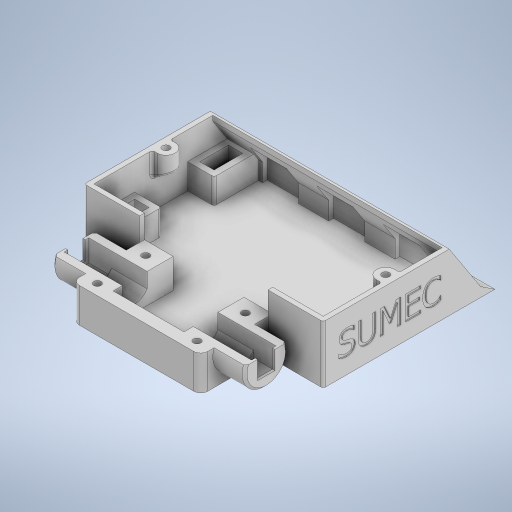
# Autodesk Inventor part: Tělo
Saved by Autodesk Inventor 2024 (Build 280153000, 153)
## iProperties
Created: 2023-04-15
Part Number: Tělo
Material: Všeobecné
Document SubType Name: Modeling
Designer: 42060
Density: 1 g/cm^3
Appearance: Výchozí
Author: 42060
Autodesk Inventor part; units mm, degrees
ref_plane "YZ Plane" through (0, 0, 0) normal (1, 0, 0) x (0, 1, 0)
ref_plane "XZ Plane" through (0, 0, 0) normal (0, 1, 0) x (-1, 0, 0)
ref_plane "XY Plane" through (0, 0, 0) normal (0, 0, 1) x (1, 0, 0)
sketch "Základ" plane through (0, 0, 0) normal (0, 0, 1) x (1, 0, 0)
  line L0 (0, 0) -> (49.75, 0)
  line L1 (49.75, 0) -> (49.75, -71.5)
  line L2 (49.75, -71.5) -> (26.75, -71.5)
  line L3 (26.75, -99.5) -> (0, -99.5)
  line L4 (0, -99.5) -> (0, 0)
  line L5 (0, -20) -> (47.75, -20)
  line L6 (47.75, -20) -> (47.75, -69.5)
  line L7 (47.75, -69.5) -> (14.75, -69.5)
  line L8 (14.75, -69.5) -> (14.75, -94.5)
  line L9 (14.75, -94.5) -> (0, -94.5)
  line L10 (26.75, -71.5) -> (26.75, -80.375)
  line L11 (26.75, -80.375) -> (26.75, -90.625)
  line L12 (26.75, -90.625) -> (26.75, -99.5)
  line L13 (26.75, -90.625) -> (14.75, -90.625)
  line L14 (26.75, -80.375) -> (14.75, -80.375)
  line L15 (26.75, -71.5) -> (26.75, -69.5)
  dimension "d0" = 49.75
  dimension "d1" = 99.5
  dimension "d3" = 2
  dimension "d5" = 28
  dimension "d14" = 10.25
  dimension "d15" = 12
  dimension "d16" = 5
  dimension "d17" = 23
  dimension "d18" = 2
  dimension "d19" = 20
  constraints: 32 end point, 8 perpendicular, 6 point on line, 3 horizontal, 2 collinear, 1 parallel, 1 vertical
  measures "d0" distance of L0.start L0.end
  measures "d1" distance between parallel lines of L3 L0
  measures "d3" distance between parallel lines of L1 L6
  measures "d5" distance of L2.end L3.start
  measures "d14" distance of L10.end L11.end
  measures "d15" distance between parallel lines of L8 L10
  measures "d16" distance between parallel lines of L9 L3
  measures "d17" distance between parallel lines of L1 L12
  measures "d18" distance between parallel lines of L2 L7
  measures "d19" distance between parallel lines of L0 L5
extrude "Podlaha" add sketch "Základ" along normal blind 2 contours L5 L6 L7 L8 L9 L4
extrude "Stěny" add sketch "Základ" along normal blind 24 contours L0 L1 L2 L15 L7 L6 L5 L4
extrude "Zadní stěny" add sketch "Základ" along normal blind 15 contours L9 L8 L13 L12 L3 L4 | L10 L14 L8 L7 L15
extrude "Stěna pod motorem" add sketch "Základ" along normal blind 5.25 contours L11 L13 L8 L14
sketch "Náčrt2" plane through (49.75, -71.5, 0) normal (1, 0, 0) x (0, 0, -1)
  line L0 (-2, 51.5) -> (-24, 51.5) projected
  line L1 (-2, 51.5) -> (-24, 51.5) projected
  line L2 (-24, 0) -> (-24, 71.5) projected
  line L3 (0, 71.5) -> (-24, 71.5) projected
  line L4 (0, 71.5) -> (0, 0) projected
  line L5 (-24, 52.5) -> (-4, 65.5)
  line L6 (-4, 65.5) -> (0, 71.5)
  dimension "d28" = 1
  dimension "d29" = 6
  dimension "d30" = 20
  constraints: 4 end point, 1 point on line
  measures "d28" distance from line of L5.start L0
  measures "d29" vertical distance of L3.start L5.end
  measures "d30" horizontal distance of L5.end L5.start
extrude "Rampa" cut sketch "Náčrt2" against normal through all
sketch "Náčrt3" plane through (0, -20, 2) normal (-1, 0, 0) x (0, 0, 1)
  line L0 (0, 0) -> (22, 0) projected
  line L1 (0, 0) -> (22, 0) projected
  line L2 (19.8687, 0) -> (7.5, 8.0396)
  line L3 (7.5, 8.0396) -> (0, 8.0396)
  line L4 (0, 8.0396) -> (0, 0)
  line L5 (22, 1) -> (2, 14) projected
  point P0 (-2, 20)
  point P1 (19.8687, 0)
  dimension "d34" = 7.5
  dimension "d37" = 2
  constraints: 6 end point, 1 horizontal, 1 parallel, 1 perpendicular, 1 point on line
  measures "d34" distance of L2.end L3.end
  measures "d37" distance between parallel lines of L2 L5
extrude "Přední rampa" cut sketch "Náčrt3" against normal up to surface (47.75 mm away)
sketch "Držák motoru" plane through (14.75, -94.5, 2) normal (-1, 0, 0) x (0, 0, 1)
  line L0 (3.25, 14.125) -> (13, 14.125) projected
  line L1 (3.25, 14.125) -> (3.25, 3.875) projected
  line L2 (3.25, 3.875) -> (13, 3.875) projected
  line L3 (6.13, 14.125) -> (12.37, 14.125)
  line L4 (12.37, 3.875) -> (6.13, 3.875)
  line L5 (3.25, 3.875) -> (13, 3.875) projected
  arc A0 (12.37, 3.875) -> (12.37, 14.125) centre (9.25, 9) ccw
  arc A1 (6.13, 14.125) -> (6.13, 3.875) centre (9.25, 9) ccw
  line L6 (15.25, 14.125) -> (15.25, 3.875) construction
  circle A2 centre (9.25, 9) radius 9
  line L7 (9.25, 18) -> (0, 18)
  line L8 (0, 0) -> (0, 82.5396) projected
  line L9 (0, 0) -> (13, 0) projected
  line L10 (13, -5) -> (13, 3.875) projected
  line L11 (0, 0) -> (13, 0) projected
  line L12 (0, 0) -> (13, 0) projected
  line L13 (12.37, 14.125) -> (12.37, 17.4419)
  line L14 (12.37, 3.875) -> (12.37, 0.5581)
  line L15 (12.37, 0.5581) -> (12.37, 0)
  line L16 (12.37, 17.4419) -> (12.37, 18)
  line L17 (12.37, 18) -> (9.25, 18)
  point P0 (-2, 94.5)
  point P1 (15.25, 9)
  point P2 (15.25, 9)
  point P3 (3.25, 9)
  point P4 (3.25, 9)
  point P5 (6.13, 3.875)
  point P6 (9.25, 0)
  point P7 (16.7333, 14)
  point P8 (16.7333, 4)
  point P9 (12.37, 0)
  dimension "d38" = 6
  dimension "d39" = 6
  dimension "d41" = 3
  dimension "d48" = 12
  constraints: 18 end point, 9 point on circle, 7 point on line, 4 tangent, 3 centre point, 3 coincident, 3 vertical, 2 horizontal alignment, 2 midpoint, 1 horizontal, 1 perpendicular
  measures "d38" radius of A0
  measures "d39" radius of A1
  measures "d41" radial gap between concentric circles of A2 A0
  measures "d48" distance between parallel lines of L1 L6
sketch "Náčrt10" plane through (14.75, -99.5, 0) normal (1, 0, 0) x (0, 0, -1)
  line L0 (-5.25, 8.875) -> (-15, 8.875) construction
  line L1 (-5.25, 8.875) -> (-17.25, 8.875) construction
  line L2 (-17.25, 8.875) -> (-17.25, 19.125) construction
  line L3 (-17.25, 19.125) -> (-5.25, 19.125) construction
  line L4 (-5.25, 19.125) -> (-5.25, 8.875) construction
  line L5 (-14.37, 8.875) -> (-8.13, 8.875)
  arc A0 (-8.13, 8.875) -> (-8.13, 19.125) centre (-11.25, 14) ccw
  line L6 (-14.37, 19.125) -> (-8.13, 19.125)
  arc A1 (-14.37, 5.5581) -> (-14.37, 22.4419) centre (-11.25, 14) ccw
  line L7 (-14.37, 8.875) -> (-14.37, 5.5581)
  line L8 (-14.37, 19.125) -> (-14.37, 22.4419)
  point P0 (0, 99.5)
  point P1 (-11.25, 19.125)
  point P2 (-11.25, 19.125)
  point P3 (-11.25, 8.875)
  point P4 (-11.25, 8.875)
  dimension "d79" = 12
  dimension "d80" = 6
  dimension "d81" = 18
  constraints: 16 end point, 5 point on line, 4 midpoint, 4 point on circle, 3 coincident, 2 centre point, 2 parallel, 2 perpendicular, 2 vertical alignment, 1 collinear, 1 horizontal, 1 horizontal alignment, 1 tangent
  measures "d79" distance between parallel lines of L4 L2
  measures "d80" radius of A0
  measures "d81" diameter of A1
extrude "Držák motoru (kulaté)" add sketch "Náčrt10" along normal blind 15
sketch "Náčrt11" plane through (29.75, -99.5, 0) normal (1, 0, 0) x (0, 0, -1)
  arc A0 (-8.13, 8.875) -> (-8.13, 19.125) centre (-11.25, 14) ccw projected
  circle A1 centre (-11.25, 14) radius 9
  line L0 (-17.25, 8.875) -> (-5.25, 8.875)
  line L1 (-5.25, 8.875) -> (-5.25, 19.125)
  line L2 (-5.25, 19.125) -> (-17.25, 19.125)
  line L3 (-17.25, 19.125) -> (-17.25, 8.875)
  line L4 (-17.25, 8.875) -> (-5.25, 19.125) construction
  line L5 (-5.25, 8.875) -> (-17.25, 19.125) construction
  line L6 (-14.37, 8.875) -> (-14.37, 5.5581) projected
  line L7 (-14.37, 22.4419) -> (-14.37, 19.125) projected
  point P0 (0, 99.5)
  dimension "d84" = 18
  constraints: 12 end point, 2 midpoint, 2 parallel, 1 centre point, 1 coincident, 1 horizontal, 1 horizontal alignment, 1 perpendicular, 1 tangent
  measures "d84" diameter of A1
extrude "Držák motoru (hranaté)" add sketch "Náčrt11" along normal blind 9.25 contours L0 L1 L2 L7 A1 L6
sketch "Náčrt7" plane through (0, 0, 2) normal (0, 0, 1) x (1, 0, 0)
  line L0 (0, -11.9604) -> (47.75, -11.9604) projected
  line L1 (0, -11.9604) -> (47.75, -11.9604) projected
  line L2 (0, 0) -> (0, -99.5) projected
  line L3 (0, -9.9604) -> (7.5, -9.9604)
  line L4 (7.5, -9.9604) -> (7.5, -16.9604)
  line L5 (7.5, -16.9604) -> (0, -16.9604)
  line L6 (0, -16.9604) -> (0, -9.9604)
  line L7 (20.125, -9.9604) -> (35.125, -9.9604)
  line L8 (35.125, -9.9604) -> (35.125, -16.9604)
  line L9 (35.125, -16.9604) -> (20.125, -16.9604)
  line L10 (20.125, -16.9604) -> (20.125, -9.9604)
  point P0 (27.625, -16.9604)
  point P1 (35.125, -11.9604)
  point P2 (20.125, -11.9604)
  point P3 (0, -16.9604)
  point P4 (7.5, -11.9604)
  dimension "d57" = 20.125
  dimension "d58" = 15
  dimension "d59" = 7.5
  dimension "d60" = 7
  dimension "d61" = 2
  constraints: 16 end point, 4 parallel, 3 point on line, 2 horizontal, 2 perpendicular, 1 midpoint
  measures "d57" horizontal distance of point (27.625, -16.96) L1.end
  measures "d58" distance of L7.start L7.end
  measures "d59" distance of L3.start L3.end
  measures "d60" distance of L7.end L8.end
  measures "d61" distance between parallel lines of L0 L3
extrude "Pření senzory" cut sketch "Náčrt7" along normal blind 15
sketch "Spodní senzory" plane through (0, 0, 2) normal (0, 0, 1) x (1, 0, 0)
  line L0 (7.5, -11.9604) -> (20.125, -11.9604) projected
  line L1 (7.5, -11.9604) -> (7.5, -9.9604) projected
  line L2 (7.5, -9.9604) -> (0, -9.9604) projected
  line L3 (0, -94.5) -> (0, -9.9604) projected
  line L4 (0, -94.5) -> (14.75, -94.5) projected
  line L5 (14.75, -94.5) -> (14.75, -69.5) projected
  line L6 (14.75, -69.5) -> (47.75, -69.5) projected
  line L7 (47.75, -69.5) -> (47.75, -11.9604) projected
  line L8 (35.125, -11.9604) -> (47.75, -11.9604) projected
  line L9 (35.125, -11.9604) -> (35.125, -9.9604) projected
  line L10 (35.125, -9.9604) -> (20.125, -9.9604) projected
  line L11 (20.125, -9.9604) -> (20.125, -11.9604) projected
  line L12 (45.25, -15.9604) -> (39.25, -15.9604)
  line L13 (39.25, -15.9604) -> (39.25, -27.9604)
  line L14 (39.25, -27.9604) -> (45.25, -27.9604)
  line L15 (45.25, -27.9604) -> (45.25, -15.9604)
  line L16 (36.75, -11.9604) -> (36.75, -30.4604)
  line L17 (36.75, -30.4604) -> (47.75, -30.4604)
  line L18 (47.75, -69.5) -> (36.75, -69.5)
  line L19 (36.75, -69.5) -> (36.75, -52.5)
  line L20 (36.75, -52.5) -> (47.75, -52.5)
  line L21 (47.75, -52.5) -> (47.75, -69.5)
  line L22 (45.25, -67) -> (39.25, -67)
  line L23 (39.25, -67) -> (39.25, -55)
  line L24 (39.25, -55) -> (45.25, -55)
  line L25 (45.25, -55) -> (45.25, -67)
  point P0 (0, 0)
  point P1 (47.75, -52.5)
  point P2 (47.75, -13.4604)
  dimension "d64" = 6
  dimension "d65" = 12
  dimension "d66" = 2.5
  dimension "d67" = 4
  dimension "d70" = 2.5
  dimension "d71" = 2.5
  dimension "d122" = 6
  dimension "d123" = 2.5
  dimension "d124" = 2.5
  dimension "d126" = 2.5
  dimension "d127" = 12
  dimension "d128" = 2.5
  constraints: 28 end point, 6 parallel, 4 perpendicular, 3 horizontal, 3 point on line, 1 vertical
  measures "d64" distance of L13.end L14.end
  measures "d65" distance of L14.end L12.start
  measures "d66" distance between parallel lines of L7 L15
  measures "d67" distance between parallel lines of L12 L8
  measures "d70" distance between parallel lines of L16 L13
  measures "d71" distance between parallel lines of L17 L14
  measures "d122" distance of L23.end L24.end
  measures "d123" distance between parallel lines of L19 L23
  measures "d124" distance between parallel lines of L7 L25
  measures "d126" distance between parallel lines of L6 L22
  measures "d127" distance of L22.end L23.end
  measures "d128" distance between parallel lines of L24 L20
extrude "Spodní senzory (díra)" cut sketch "Spodní senzory" against normal through all contours L15 L14 L13 L12 | L22 L23 L24 L25
extrude "Spodní senzory zvýšení" add sketch "Spodní senzory" along normal blind 10.5 contours L8 L7 L17 L16 | L19 L20 L7 L6
sketch "Náčrt12" plane through (0, 0, 15) normal (0, 0, 1) x (1, 0, 0)
  line L0 (26.75, -80.375) -> (26.75, -71.5) projected
  line L1 (26.75, -69.5) -> (26.75, -71.5) projected
  line L2 (26.75, -69.5) -> (14.75, -69.5) projected
  line L3 (14.75, -69.5) -> (14.75, -80.375) projected
  line L4 (14.75, -80.375) -> (26.75, -80.375) projected
  line L5 (26.75, -99.5) -> (26.75, -90.625) projected
  line L6 (26.75, -90.625) -> (14.75, -90.625) projected
  line L7 (14.75, -90.625) -> (14.75, -94.5) projected
  line L8 (14.75, -94.5) -> (0, -94.5) projected
  line L9 (0, -94.5) -> (0, -99.5) projected
  line L10 (0, -99.5) -> (26.75, -99.5) projected
  point P0 (0, 0)
extrude "Vyrovnání držáku motoru" cut sketch "Náčrt12" against normal up to surface (0.63 mm away)
sketch "Náčrt13" plane through (14.75, -80.375, 14.37) normal (0, 0, 1) x (1, 0, 0)
  line L0 (0, 0) -> (0, 10.875) projected
  line L1 (0, 10.875) -> (12, 10.875) projected
  line L2 (0, -14.125) -> (0, -10.25) projected
  line L3 (0, -10.25) -> (24.25, -10.25) projected
  point P0 (-14.75, 80.375)
  point P1 (6, 5.4375)
  point P2 (6, -14.6875)
  dimension "d89" = 6
  dimension "d90" = 5.4375
  dimension "d91" = 6
  dimension "d92" = 4.4375
  measures "d89" distance from line of L0 point (6, 5.438)
  measures "d90" distance from line of L1 point (6, 5.438)
  measures "d91" distance from line of L2 point (6, -14.687)
  measures "d92" distance from line of L3 point (6, -14.687)
hole "Díry pro objímku motoru" at (20.75, -95.0625, 14.37) at (20.75, -74.9375, 14.37) direction (0, 0, -1) diameter 3 depth 6
fillet "Zaoblení1" radius 3 1 edges at (26.75, -99.5, 7.185)
fillet "Zaoblení2" radius 1 3 edges at (49.75, -71.5, 12) (36.75, -30.4604, 7.25) (36.75, -52.5, 7.25)
sketch "Náčrt14" plane through (39, -99.5, 0) normal (1, 0, 0) x (0, 0, -1)
  line L0 (-14.37, 19.125) -> (-5.25, 19.125) projected
  line L1 (-5.25, 19.125) -> (-5.25, 8.875) projected
  line L2 (-5.25, 8.875) -> (-14.37, 8.875) projected
  line L3 (-14.37, 8.875) -> (-14.37, 5.5581) projected
  arc A0 (-14.37, 5.5581) -> (-14.37, 22.4419) centre (-11.25, 14) ccw projected
  line L4 (-14.37, 22.4419) -> (-14.37, 19.125) projected
  line L5 (-14.37, 10.375) -> (-6.75, 10.375)
  line L6 (-6.75, 10.375) -> (-6.75, 17.625)
  line L7 (-6.75, 17.625) -> (-14.37, 17.625)
  line L8 (-14.37, 8.875) -> (-14.37, 10.375)
  line L9 (-14.37, 17.625) -> (-14.37, 19.125)
  point P0 (0, 99.5)
  dimension "d108" = 1.5
  dimension "d109" = 1.5
  dimension "d110" = 1.5
  constraints: 10 end point, 2 perpendicular, 2 point on line, 2 vertical, 2 vertical alignment
  measures "d108" distance between parallel lines of L5 L2
  measures "d109" distance between parallel lines of L1 L6
  measures "d110" distance between parallel lines of L0 L7
extrude "Vysunutí19" add sketch "Náčrt14" along normal blind 1
chamfer "Zkosení1" distance 1 angle 45 1 edges at (40, -85.5, 2.25)
chamfer "Zkosení2" distance 0.25 angle 45 2 edges at (29.75, -88.4394, 6.0193) (29.75, -82.5606, 6.0193)
sketch "Náčrt16" plane through (0, 0, 24) normal (0, 0, 1) x (1, 0, 0)
  line L0 (47.75, -52.5) -> (47.75, -30.4604) projected
  line L1 (47.75, -37.7302) -> (45.75, -37.7302)
  arc A0 (45.75, -37.7302) -> (45.75, -45.2302) centre (45.75, -41.4802) ccw
  line L2 (45.75, -45.2302) -> (47.75, -45.2302)
  point P0 (0, 0)
  point P1 (47.75, -41.4802)
  dimension "d130" = 3.75
  dimension "d131" = 2
  constraints: 4 end point, 2 point on circle, 2 point on line, 2 tangent, 1 centre point, 1 horizontal, 1 horizontal alignment, 1 midpoint, 1 parallel
  measures "d130" radius of A0
  measures "d131" distance of L2.start L2.end
extrude "Vysunutí20" add sketch "Náčrt16" against normal blind 10
sketch "Náčrt17" plane through (0, 0, 24) normal (0, 0, 1) x (1, 0, 0)
  arc A0 (45.75, -37.7302) -> (45.75, -45.2302) centre (45.75, -41.4802) ccw projected
  point P0 (0, 0)
  constraints: 1 coincident
hole "Díra2" at (45.75, -41.4802, 24) direction (0, 0, -1) diameter 3 depth 6
sketch "Náčrt18" plane through (45.75, -45.2302, 24) normal (0, -1, 0) x (1, 0, 0)
  line L0 (-10.625, -22) -> (-25.625, -22) projected
  line L1 (-3.75, -10) -> (0, -10) projected
  line L2 (0, -10) -> (2, -10) projected
  line L3 (-3.75, 0) -> (-3.75, -10) projected
  line L4 (-3.75, -6.6802) -> (2, -10)
  point P0 (-45.75, -24)
  dimension "d141" = 30
  constraints: 2 end point, 1 point on line
  measures "d141" angle of L1 L4
extrude "Vysunutí21" cut sketch "Náčrt18" against normal blind 10
fillet "Zaoblení3" radius 1 7 edges at (46.75, -45.2302, 14.5774) (46.75, -37.7302, 14.5774) (43.0983, -44.1318, 16.6856) (43.0983, -38.8285, 16.6856) (47.75, -45.2302, 19) (47.75, -37.7302, 19) (47.75, -41.4802, 14)
mirror "Zrcadlení těla" about plane through (0, 0, 0) normal (1, 0, 0)
sketch "Náčrt15" plane through (49.75, -70.5, 0) normal (1, 0, 0) x (0, 0, -1)
  line L0 (-17, 5) -> (-17, 50) construction
  line L1 (-17, 50) -> (-6, 50) construction
  line L2 (-6, 50) -> (-6, 5) construction
  line L3 (-6, 5) -> (-17, 5) construction
  line L4 (-24, -1) -> (0, -1) projected
  line L5 (0, 0) -> (0, 70.5) projected
  spline S0 degree 2 poles (-6.6434, 8.8006) (-6.6434, 7.7147) (-7.0972, 6.1912) (-7.4214, 5.5186) knots 0 0 0 1 2 2 2
  line L6 (-7.4214, 5.5186) -> (-9.0908, 5.5186)
  line L7 (-9.0908, 5.5186) -> (-9.0908, 5.6159)
  spline S1 degree 2 poles (-9.0908, 5.6159) (-8.4749, 6.2723) (-7.7942, 7.9335) (-7.7942, 8.7034) knots 0 0 0 1 2 2 2
  spline S2 degree 2 poles (-7.7942, 8.7034) (-7.7942, 9.8055) (-8.7099, 10.9319) (-9.4635, 10.9319) knots 0 0 0 1 2 2 2
  spline S3 degree 2 poles (-9.4635, 10.9319) (-10.0632, 10.9319) (-10.8088, 10.3404) (-10.9951, 9.7002) knots 0 0 0 1 2 2 2
  spline S4 degree 2 poles (-10.9951, 9.7002) (-11.1248, 9.2382) (-11.3031, 8.4684) (-11.4489, 7.893) knots 0 0 0 1 2 2 2
  spline S5 degree 2 poles (-11.4489, 7.893) (-11.5867, 7.3744) (-12, 6.5559) (-12.3323, 6.2399) knots 0 0 0 1 2 2 2
  spline S6 degree 2 poles (-12.3323, 6.2399) (-12.6645, 5.9319) (-13.5559, 5.5916) (-14.1394, 5.5916) knots 0 0 0 1 2 2 2
  spline S7 degree 2 poles (-14.1394, 5.5916) (-15.3549, 5.5916) (-17, 7.4878) (-17, 8.9546) knots 0 0 0 1 2 2 2
  spline S8 degree 2 poles (-17, 8.9546) (-17, 9.7974) (-16.6677, 11.2885) (-16.3517, 11.9287) knots 0 0 0 1 2 2 2
  line L8 (-16.3517, 11.9287) -> (-14.7634, 11.9287)
  line L9 (-14.7634, 11.9287) -> (-14.7634, 11.8314)
  spline S9 degree 2 poles (-14.7634, 11.8314) (-15.201, 11.3533) (-15.8493, 9.8622) (-15.8493, 9.0438) knots 0 0 0 1 2 2 2
  spline S10 degree 2 poles (-15.8493, 9.0438) (-15.8493, 8.1199) (-14.9822, 6.9773) (-14.2771, 6.9773) knots 0 0 0 1 2 2 2
  spline S11 degree 2 poles (-14.2771, 6.9773) (-13.6451, 6.9773) (-12.8914, 7.6499) (-12.7212, 8.282) knots 0 0 0 1 2 2 2
  spline S12 degree 2 poles (-12.7212, 8.282) (-12.6078, 8.7034) (-12.316, 9.9271) (-12.1945, 10.3323) knots 0 0 0 1 2 2 2
  spline S13 degree 2 poles (-12.1945, 10.3323) (-11.8784, 11.3614) (-10.6062, 12.3177) (-9.6742, 12.3177) knots 0 0 0 1 2 2 2
  spline S14 degree 2 poles (-9.6742, 12.3177) (-9.0827, 12.3177) (-7.9481, 11.8395) (-7.5511, 11.41) knots 0 0 0 1 2 2 2
  spline S15 degree 2 poles (-7.5511, 11.41) (-7.1135, 10.9319) (-6.6434, 9.7164) (-6.6434, 8.8006) knots 0 0 0 1 2 2 2
  spline S16 degree 2 poles (-6.611, 17.1637) (-6.611, 16.2804) (-7.0729, 14.9676) (-7.5348, 14.5057) knots 0 0 0 1 2 2 2
  spline S17 degree 2 poles (-7.5348, 14.5057) (-8.0535, 13.9789) (-9.5122, 13.5494) (-10.5818, 13.5494) knots 0 0 0 1 2 2 2
  line L10 (-10.5818, 13.5494) -> (-16.8217, 13.5494)
  line L11 (-16.8217, 13.5494) -> (-16.8217, 14.8784)
  line L12 (-16.8217, 14.8784) -> (-10.5818, 14.8784)
  spline S18 degree 2 poles (-10.5818, 14.8784) (-9.8849, 14.8784) (-8.9449, 15.0567) (-8.564, 15.3079) knots 0 0 0 1 2 2 2
  spline S19 degree 2 poles (-8.564, 15.3079) (-8.1588, 15.5754) (-7.7455, 16.4992) (-7.7455, 17.1637) knots 0 0 0 1 2 2 2
  spline S20 degree 2 poles (-7.7455, 17.1637) (-7.7455, 17.7877) (-8.1588, 18.7601) (-8.564, 19.0276) knots 0 0 0 1 2 2 2
  spline S21 degree 2 poles (-8.564, 19.0276) (-8.9449, 19.2788) (-9.8768, 19.4571) (-10.5494, 19.4571) knots 0 0 0 1 2 2 2
  line L13 (-10.5494, 19.4571) -> (-16.8217, 19.4571)
  line L14 (-16.8217, 19.4571) -> (-16.8217, 20.7861)
  line L15 (-16.8217, 20.7861) -> (-10.5818, 20.7861)
  spline S22 degree 2 poles (-10.5818, 20.7861) (-9.5365, 20.7861) (-8.0454, 20.3647) (-7.5348, 19.8298) knots 0 0 0 1 2 2 2
  spline S23 degree 2 poles (-7.5348, 19.8298) (-7.0648, 19.3517) (-6.611, 18.0875) (-6.611, 17.1637) knots 0 0 0 1 2 2 2
  line L16 (-6.8217, 31.2642) -> (-6.8217, 29.9352)
  line L17 (-6.8217, 29.9352) -> (-15.436, 29.9352)
  line L18 (-15.436, 29.9352) -> (-9.577, 27.3258)
  line L19 (-9.577, 27.3258) -> (-9.577, 26.5154)
  line L20 (-9.577, 26.5154) -> (-15.436, 23.9303)
  line L21 (-15.436, 23.9303) -> (-6.8217, 23.9303)
  line L22 (-6.8217, 23.9303) -> (-6.8217, 22.6904)
  line L23 (-6.8217, 22.6904) -> (-16.8217, 22.6904)
  line L24 (-16.8217, 22.6904) -> (-16.8217, 24.5057)
  line L25 (-16.8217, 24.5057) -> (-11.2545, 27.0016)
  line L26 (-11.2545, 27.0016) -> (-16.8217, 29.4165)
  line L27 (-16.8217, 29.4165) -> (-16.8217, 31.2642)
  line L28 (-16.8217, 31.2642) -> (-6.8217, 31.2642)
  line L29 (-6.8217, 33.2901) -> (-16.8217, 33.2901)
  line L30 (-16.8217, 33.2901) -> (-16.8217, 39.5462)
  line L31 (-16.8217, 39.5462) -> (-15.6386, 39.5462)
  line L32 (-15.6386, 39.5462) -> (-15.6386, 34.6191)
  line L33 (-15.6386, 34.6191) -> (-12.8995, 34.6191)
  line L34 (-12.8995, 34.6191) -> (-12.8995, 39.2139)
  line L35 (-12.8995, 39.2139) -> (-11.7164, 39.2139)
  line L36 (-11.7164, 39.2139) -> (-11.7164, 34.6191)
  line L37 (-11.7164, 34.6191) -> (-8.0049, 34.6191)
  line L38 (-8.0049, 34.6191) -> (-8.0049, 39.5462)
  line L39 (-8.0049, 39.5462) -> (-6.8217, 39.5462)
  line L40 (-6.8217, 39.5462) -> (-6.8217, 33.2901)
  spline S24 degree 2 poles (-6.6434, 44.9109) (-6.6434, 43.9384) (-7.2998, 42.2934) (-7.9562, 41.6937) knots 0 0 0 1 2 2 2
  spline S25 degree 2 poles (-7.9562, 41.6937) (-8.6045, 41.094) (-10.5494, 40.4376) (-11.8136, 40.4376) knots 0 0 0 1 2 2 2
  spline S26 degree 2 poles (-11.8136, 40.4376) (-13.0697, 40.4376) (-14.9335, 41.0778) (-15.6224, 41.6856) knots 0 0 0 1 2 2 2
  spline S27 degree 2 poles (-15.6224, 41.6856) (-16.295, 42.2853) (-17, 43.9222) (-17, 44.9352) knots 0 0 0 1 2 2 2
  spline S28 degree 2 poles (-17, 44.9352) (-17, 45.4376) (-16.8541, 46.3209) (-16.7407, 46.6937) knots 0 0 0 1 2 2 2
  spline S29 degree 2 poles (-16.7407, 46.6937) (-16.6353, 47.0178) (-16.3355, 47.6904) (-16.1572, 48.0227) knots 0 0 0 1 2 2 2
  line L41 (-16.1572, 48.0227) -> (-14.5527, 48.0227)
  line L42 (-14.5527, 48.0227) -> (-14.5527, 47.9173)
  spline S30 degree 2 poles (-14.5527, 47.9173) (-14.7147, 47.7391) (-15.1686, 47.188) (-15.3874, 46.7909) knots 0 0 0 1 2 2 2
  spline S31 degree 2 poles (-15.3874, 46.7909) (-15.5981, 46.41) (-15.8655, 45.5105) (-15.8655, 44.9271) knots 0 0 0 1 2 2 2
  spline S32 degree 2 poles (-15.8655, 44.9271) (-15.8655, 44.2869) (-15.3387, 43.1442) (-14.8363, 42.7147) knots 0 0 0 1 2 2 2
  spline S33 degree 2 poles (-14.8363, 42.7147) (-14.3258, 42.2934) (-12.778, 41.8233) (-11.8136, 41.8233) knots 0 0 0 1 2 2 2
  spline S34 degree 2 poles (-11.8136, 41.8233) (-10.7844, 41.8233) (-9.3015, 42.3177) (-8.7909, 42.7472) knots 0 0 0 1 2 2 2
  spline S35 degree 2 poles (-8.7909, 42.7472) (-8.2966, 43.1686) (-7.7942, 44.295) (-7.7942, 44.9271) knots 0 0 0 1 2 2 2
  spline S36 degree 2 poles (-7.7942, 44.9271) (-7.7942, 45.5024) (-8.0778, 46.483) (-8.2885, 46.8639) knots 0 0 0 1 2 2 2
  spline S37 degree 2 poles (-8.2885, 46.8639) (-8.4992, 47.2285) (-8.9368, 47.7715) (-9.0908, 47.9254) knots 0 0 0 1 2 2 2
  line L43 (-9.0908, 47.9254) -> (-9.0908, 48.0227)
  line L44 (-9.0908, 48.0227) -> (-7.5024, 48.0227)
  spline S38 degree 2 poles (-7.5024, 48.0227) (-7.3485, 47.6904) (-7.0648, 47.107) (-6.9352, 46.6937) knots 0 0 0 1 2 2 2
  spline S39 degree 2 poles (-6.9352, 46.6937) (-6.7893, 46.2561) (-6.6434, 45.5105) (-6.6434, 44.9109) knots 0 0 0 1 2 2 2
  dimension "d145" = 11
  dimension "d146" = 45
  dimension "d147" = 6
  dimension "d148" = 6
  constraints: 2 other
  measures "d145" distance of L0.end L1.end
  measures "d146" distance of L1.end L2.end
  measures "d147" distance between parallel lines of L3 L4
  measures "d148" distance between parallel lines of L5 L2
emboss "Reliéf1" sketch "Náčrt15" operation cut depth 0.4 direction (-1, 0, 0)
sketch "Náčrt19" plane through (-49.75, -70.5, 0) normal (-1, 0, 0) x (0, 0, 1)
  line L0 (17, 50) -> (17, 5) construction
  line L1 (17, 5) -> (6, 5) construction
  line L2 (6, 5) -> (6, 50) construction
  line L3 (6, 50) -> (17, 50) construction
  line L4 (24, -1) -> (0, -1) projected
  line L5 (0, 0) -> (0, 70.5) projected
  spline S0 degree 2 poles (6.6434, 46.1994) (6.6434, 47.2853) (7.0972, 48.8088) (7.4214, 49.4814) knots 0 0 0 1 2 2 2
  line L6 (7.4214, 49.4814) -> (9.0908, 49.4814)
  line L7 (9.0908, 49.4814) -> (9.0908, 49.3841)
  spline S1 degree 2 poles (9.0908, 49.3841) (8.4749, 48.7277) (7.7942, 47.0665) (7.7942, 46.2966) knots 0 0 0 1 2 2 2
  spline S2 degree 2 poles (7.7942, 46.2966) (7.7942, 45.1945) (8.7099, 44.0681) (9.4635, 44.0681) knots 0 0 0 1 2 2 2
  spline S3 degree 2 poles (9.4635, 44.0681) (10.0632, 44.0681) (10.8088, 44.6596) (10.9951, 45.2998) knots 0 0 0 1 2 2 2
  spline S4 degree 2 poles (10.9951, 45.2998) (11.1248, 45.7618) (11.3031, 46.5316) (11.4489, 47.107) knots 0 0 0 1 2 2 2
  spline S5 degree 2 poles (11.4489, 47.107) (11.5867, 47.6256) (12, 48.4441) (12.3323, 48.7601) knots 0 0 0 1 2 2 2
  spline S6 degree 2 poles (12.3323, 48.7601) (12.6645, 49.0681) (13.5559, 49.4084) (14.1394, 49.4084) knots 0 0 0 1 2 2 2
  spline S7 degree 2 poles (14.1394, 49.4084) (15.3549, 49.4084) (17, 47.5122) (17, 46.0454) knots 0 0 0 1 2 2 2
  spline S8 degree 2 poles (17, 46.0454) (17, 45.2026) (16.6677, 43.7115) (16.3517, 43.0713) knots 0 0 0 1 2 2 2
  line L8 (16.3517, 43.0713) -> (14.7634, 43.0713)
  line L9 (14.7634, 43.0713) -> (14.7634, 43.1686)
  spline S9 degree 2 poles (14.7634, 43.1686) (15.201, 43.6467) (15.8493, 45.1378) (15.8493, 45.9562) knots 0 0 0 1 2 2 2
  spline S10 degree 2 poles (15.8493, 45.9562) (15.8493, 46.8801) (14.9822, 48.0227) (14.2771, 48.0227) knots 0 0 0 1 2 2 2
  spline S11 degree 2 poles (14.2771, 48.0227) (13.6451, 48.0227) (12.8914, 47.3501) (12.7212, 46.718) knots 0 0 0 1 2 2 2
  spline S12 degree 2 poles (12.7212, 46.718) (12.6078, 46.2966) (12.316, 45.0729) (12.1945, 44.6677) knots 0 0 0 1 2 2 2
  spline S13 degree 2 poles (12.1945, 44.6677) (11.8784, 43.6386) (10.6062, 42.6823) (9.6742, 42.6823) knots 0 0 0 1 2 2 2
  spline S14 degree 2 poles (9.6742, 42.6823) (9.0827, 42.6823) (7.9481, 43.1605) (7.5511, 43.59) knots 0 0 0 1 2 2 2
  spline S15 degree 2 poles (7.5511, 43.59) (7.1135, 44.0681) (6.6434, 45.2836) (6.6434, 46.1994) knots 0 0 0 1 2 2 2
  spline S16 degree 2 poles (6.611, 37.8363) (6.611, 38.7196) (7.0729, 40.0324) (7.5348, 40.4943) knots 0 0 0 1 2 2 2
  spline S17 degree 2 poles (7.5348, 40.4943) (8.0535, 41.0211) (9.5122, 41.4506) (10.5818, 41.4506) knots 0 0 0 1 2 2 2
  line L10 (10.5818, 41.4506) -> (16.8217, 41.4506)
  line L11 (16.8217, 41.4506) -> (16.8217, 40.1216)
  line L12 (16.8217, 40.1216) -> (10.5818, 40.1216)
  spline S18 degree 2 poles (10.5818, 40.1216) (9.8849, 40.1216) (8.9449, 39.9433) (8.564, 39.6921) knots 0 0 0 1 2 2 2
  spline S19 degree 2 poles (8.564, 39.6921) (8.1588, 39.4246) (7.7455, 38.5008) (7.7455, 37.8363) knots 0 0 0 1 2 2 2
  spline S20 degree 2 poles (7.7455, 37.8363) (7.7455, 37.2123) (8.1588, 36.2399) (8.564, 35.9724) knots 0 0 0 1 2 2 2
  spline S21 degree 2 poles (8.564, 35.9724) (8.9449, 35.7212) (9.8768, 35.5429) (10.5494, 35.5429) knots 0 0 0 1 2 2 2
  line L13 (10.5494, 35.5429) -> (16.8217, 35.5429)
  line L14 (16.8217, 35.5429) -> (16.8217, 34.2139)
  line L15 (16.8217, 34.2139) -> (10.5818, 34.2139)
  spline S22 degree 2 poles (10.5818, 34.2139) (9.5365, 34.2139) (8.0454, 34.6353) (7.5348, 35.1702) knots 0 0 0 1 2 2 2
  spline S23 degree 2 poles (7.5348, 35.1702) (7.0648, 35.6483) (6.611, 36.9125) (6.611, 37.8363) knots 0 0 0 1 2 2 2
  line L16 (6.8217, 23.7358) -> (6.8217, 25.0648)
  line L17 (6.8217, 25.0648) -> (15.436, 25.0648)
  line L18 (15.436, 25.0648) -> (9.577, 27.6742)
  line L19 (9.577, 27.6742) -> (9.577, 28.4846)
  line L20 (9.577, 28.4846) -> (15.436, 31.0697)
  line L21 (15.436, 31.0697) -> (6.8217, 31.0697)
  line L22 (6.8217, 31.0697) -> (6.8217, 32.3096)
  line L23 (6.8217, 32.3096) -> (16.8217, 32.3096)
  line L24 (16.8217, 32.3096) -> (16.8217, 30.4943)
  line L25 (16.8217, 30.4943) -> (11.2545, 27.9984)
  line L26 (11.2545, 27.9984) -> (16.8217, 25.5835)
  line L27 (16.8217, 25.5835) -> (16.8217, 23.7358)
  line L28 (16.8217, 23.7358) -> (6.8217, 23.7358)
  line L29 (6.8217, 21.7099) -> (16.8217, 21.7099)
  line L30 (16.8217, 21.7099) -> (16.8217, 15.4538)
  line L31 (16.8217, 15.4538) -> (15.6386, 15.4538)
  line L32 (15.6386, 15.4538) -> (15.6386, 20.3809)
  line L33 (15.6386, 20.3809) -> (12.8995, 20.3809)
  line L34 (12.8995, 20.3809) -> (12.8995, 15.7861)
  line L35 (12.8995, 15.7861) -> (11.7164, 15.7861)
  line L36 (11.7164, 15.7861) -> (11.7164, 20.3809)
  line L37 (11.7164, 20.3809) -> (8.0049, 20.3809)
  line L38 (8.0049, 20.3809) -> (8.0049, 15.4538)
  line L39 (8.0049, 15.4538) -> (6.8217, 15.4538)
  line L40 (6.8217, 15.4538) -> (6.8217, 21.7099)
  spline S24 degree 2 poles (6.6434, 10.0891) (6.6434, 11.0616) (7.2998, 12.7066) (7.9562, 13.3063) knots 0 0 0 1 2 2 2
  spline S25 degree 2 poles (7.9562, 13.3063) (8.6045, 13.906) (10.5494, 14.5624) (11.8136, 14.5624) knots 0 0 0 1 2 2 2
  spline S26 degree 2 poles (11.8136, 14.5624) (13.0697, 14.5624) (14.9335, 13.9222) (15.6224, 13.3144) knots 0 0 0 1 2 2 2
  spline S27 degree 2 poles (15.6224, 13.3144) (16.295, 12.7147) (17, 11.0778) (17, 10.0648) knots 0 0 0 1 2 2 2
  spline S28 degree 2 poles (17, 10.0648) (17, 9.5624) (16.8541, 8.6791) (16.7407, 8.3063) knots 0 0 0 1 2 2 2
  spline S29 degree 2 poles (16.7407, 8.3063) (16.6353, 7.9822) (16.3355, 7.3096) (16.1572, 6.9773) knots 0 0 0 1 2 2 2
  line L41 (16.1572, 6.9773) -> (14.5527, 6.9773)
  line L42 (14.5527, 6.9773) -> (14.5527, 7.0827)
  spline S30 degree 2 poles (14.5527, 7.0827) (14.7147, 7.2609) (15.1686, 7.812) (15.3874, 8.2091) knots 0 0 0 1 2 2 2
  spline S31 degree 2 poles (15.3874, 8.2091) (15.5981, 8.59) (15.8655, 9.4895) (15.8655, 10.0729) knots 0 0 0 1 2 2 2
  spline S32 degree 2 poles (15.8655, 10.0729) (15.8655, 10.7131) (15.3387, 11.8558) (14.8363, 12.2853) knots 0 0 0 1 2 2 2
  spline S33 degree 2 poles (14.8363, 12.2853) (14.3258, 12.7066) (12.778, 13.1767) (11.8136, 13.1767) knots 0 0 0 1 2 2 2
  spline S34 degree 2 poles (11.8136, 13.1767) (10.7844, 13.1767) (9.3015, 12.6823) (8.7909, 12.2528) knots 0 0 0 1 2 2 2
  spline S35 degree 2 poles (8.7909, 12.2528) (8.2966, 11.8314) (7.7942, 10.705) (7.7942, 10.0729) knots 0 0 0 1 2 2 2
  spline S36 degree 2 poles (7.7942, 10.0729) (7.7942, 9.4976) (8.0778, 8.517) (8.2885, 8.1361) knots 0 0 0 1 2 2 2
  spline S37 degree 2 poles (8.2885, 8.1361) (8.4992, 7.7715) (8.9368, 7.2285) (9.0908, 7.0746) knots 0 0 0 1 2 2 2
  line L43 (9.0908, 7.0746) -> (9.0908, 6.9773)
  line L44 (9.0908, 6.9773) -> (7.5024, 6.9773)
  spline S38 degree 2 poles (7.5024, 6.9773) (7.3485, 7.3096) (7.0648, 7.893) (6.9352, 8.3063) knots 0 0 0 1 2 2 2
  spline S39 degree 2 poles (6.9352, 8.3063) (6.7893, 8.7439) (6.6434, 9.4895) (6.6434, 10.0891) knots 0 0 0 1 2 2 2
  dimension "d149" = 11
  dimension "d150" = 45
  dimension "d151" = 6
  dimension "d152" = 6
  constraints: 2 other
  measures "d149" distance of L0.end L1.end
  measures "d150" distance of L1.end L2.end
  measures "d151" distance between parallel lines of L4 L1
  measures "d152" distance between parallel lines of L5 L2
emboss "Reliéf2" sketch "Náčrt19" operation cut depth 0.4 direction (1, 0, 0)
